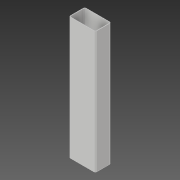
# Autodesk Inventor part: Perfil 30x501
Saved by Autodesk Inventor 2019 (Build 230136000, 136)
## iProperties
Created: 2019-11-05
Part Number: Perfil 30x501
Material: Generic
Document SubType Name: Modeling
Designer: Charlie
Density: 1 g/cm^3
Appearance: Default
Author: Charlie
Autodesk Inventor part; units mm, degrees
ref_plane "YZ Plane" through (0, 0, 0) normal (1, 0, 0) x (0, 1, 0)
ref_plane "XZ Plane" through (0, 0, 0) normal (0, 1, 0) x (-1, 0, 0)
ref_plane "XY Plane" through (0, 0, 0) normal (0, 0, 1) x (1, 0, 0)
sketch "Sketch1" plane through (0, 0, 0) normal (0, 1, 0) x (-1, 0, 0)
  line L0 (25, 15) -> (-25, 15)
  line L1 (-25, 15) -> (-25, -15)
  line L2 (-25, -15) -> (25, -15)
  line L3 (25, -15) -> (25, 15)
  line L4 (25, 15) -> (-25, -15) construction
  line L5 (-25, 15) -> (25, -15) construction
  point P0 (0, 0)
  dimension "d0" = 50
  dimension "d1" = 30
  constraints: 12 end point, 2 midpoint, 2 parallel, 1 horizontal, 1 perpendicular
  measures "d0" distance of L2.end L1.end
  measures "d1" distance of L1.end L0.end
extrude "Extrusion1" add sketch "Sketch1" along normal mid plane 230
fillet "Fillet1" radius 3 4 edges at (25, 0, 15) (25, 0, -15) (-25, 0, 15) (-25, 0, -15)
shell "Shell1" thickness 1.2 removed faces 2 at (-7.3333, 115, -5) at (-7.3333, -115, -5)
body "Solid1"
